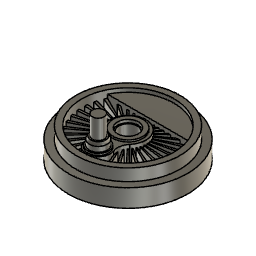
Leading Wheel (Autodesk Fusion 360 design; units mm, degrees)
Autodesk Fusion 360 part; units mm, degrees
sketch "Sketch1" plane through (0, 0, 0) normal (0, 0, 1) x (1, 0, 0) in component "Component"
  circle A0 centre (0, 0) radius 1.55
  circle A1 centre (0, 0) radius 1.75
  circle A2 centre (0, 0) radius 2.5
  circle A3 centre (0, 0) radius 10
  circle A4 centre (0, 0) radius 8.75
  arc A5 (2.2613, -1.9714) -> (1.8622, -4.2706) centre (3.9573, -3.45) ccw
  arc A6 (-1.8622, -4.2706) -> (-2.2613, -1.9714) centre (-3.9573, -3.45) ccw
  circle A7 centre (0, 0) radius 7.75
  arc A8 (2.2613, -1.9714) -> (-2.2613, -1.9714) centre (0, 0) ccw
  arc A9 (-1.8622, -4.2706) -> (1.8622, -4.2706) centre (0, -5) ccw
  line L0 (-0.1744, 2.9949) -> (-0.2026, 3.4782)
  line L1 (-0.3483, 2.9797) -> (-0.4065, 3.4782)
  line L2 (-0.6918, 2.9191) -> (-0.8243, 3.4782)
  line L3 (-0.8604, 2.874) -> (-1.0413, 3.4782)
  line L4 (-1.1882, 2.7546) -> (-1.5003, 3.4782)
  line L5 (-1.3464, 2.6809) -> (-1.7468, 3.4782)
  line L6 (-1.6485, 2.5065) -> (-2.2876, 3.4782)
  line L7 (-1.7915, 2.4064) -> (-2.5894, 3.4782)
  line L8 (-2.0587, 2.1821) -> (-3.2815, 3.4782)
  line L9 (-2.1821, 2.0587) -> (-3.6867, 3.4782)
  line L10 (-2.4064, 1.7915) -> (-4.672, 3.4782)
  line L11 (-2.5065, 1.6485) -> (-5.2883, 3.4782)
  line L12 (-2.6809, 1.3464) -> (-6.9257, 3.4782)
  line L13 (-2.7546, 1.1882) -> (-7.1162, 3.0696)
  line L14 (-2.874, 0.8604) -> (-7.4244, 2.2227)
  line L15 (-2.9191, 0.6918) -> (-7.5411, 1.7873)
  line L16 (-2.9797, 0.3483) -> (-7.6976, 0.8997)
  line L17 (-2.9949, 0.1744) -> (-7.7369, 0.4506)
  line L18 (-2.9949, -0.1744) -> (-7.7369, -0.4506)
  line L19 (-2.9797, -0.3483) -> (-7.6976, -0.8997)
  line L20 (-2.9191, -0.6918) -> (-7.5411, -1.7873)
  line L21 (-2.874, -0.8604) -> (-7.4244, -2.2227)
  line L22 (-2.7546, -1.1882) -> (-7.1162, -3.0696)
  line L23 (-2.6809, -1.3464) -> (-6.9257, -3.4782)
  line L24 (-2.5065, -1.6485) -> (-6.475, -4.2587)
  line L25 (-2.4064, -1.7915) -> (-6.2165, -4.628)
  line L26 (-2.1861, -2.0624) -> (-5.6371, -5.3184)
  line L27 (-2.082, -2.2067) -> (-5.3184, -5.6371)
  line L28 (-1.8963, -2.5472) -> (-4.628, -6.2165)
  line L29 (-1.8156, -2.7604) -> (-4.2587, -6.475)
  line L30 (-1.7078, -3.4005) -> (-3.4782, -6.9257)
  line L31 (-1.9291, -4.4721) -> (-3.0696, -7.1162)
  line L32 (-1.7736, -5.9243) -> (-2.2227, -7.4244)
  line L33 (-1.4989, -6.3242) -> (-1.7873, -7.5411)
  line L34 (-0.7987, -6.8336) -> (-0.8997, -7.6976)
  line L35 (-0.4053, -6.9585) -> (-0.4506, -7.7369)
  line L36 (0.4053, -6.9585) -> (0.4506, -7.7369)
  line L37 (0.7987, -6.8336) -> (0.8997, -7.6976)
  line L38 (1.4989, -6.3242) -> (1.7873, -7.5411)
  line L39 (1.7736, -5.9243) -> (2.2227, -7.4244)
  line L40 (1.9291, -4.4721) -> (3.0696, -7.1162)
  line L41 (1.7078, -3.4005) -> (3.4782, -6.9257)
  line L42 (1.8156, -2.7604) -> (4.2587, -6.475)
  line L43 (1.8963, -2.5472) -> (4.628, -6.2165)
  line L44 (2.082, -2.2067) -> (5.3184, -5.6371)
  line L45 (2.1861, -2.0624) -> (5.6371, -5.3184)
  line L46 (2.4064, -1.7915) -> (6.2165, -4.628)
  line L47 (2.5065, -1.6485) -> (6.475, -4.2587)
  line L48 (2.6809, -1.3464) -> (6.9257, -3.4782)
  line L49 (2.7546, -1.1882) -> (7.1162, -3.0696)
  line L50 (2.874, -0.8604) -> (7.4244, -2.2227)
  line L51 (2.9191, -0.6918) -> (7.5411, -1.7873)
  line L52 (2.9797, -0.3483) -> (7.6976, -0.8997)
  line L53 (2.9949, -0.1744) -> (7.7369, -0.4506)
  line L54 (2.9949, 0.1744) -> (7.7369, 0.4506)
  line L55 (2.9797, 0.3483) -> (7.6976, 0.8997)
  line L56 (2.9191, 0.6918) -> (7.5411, 1.7873)
  line L57 (2.874, 0.8604) -> (7.4244, 2.2227)
  line L58 (2.7546, 1.1882) -> (7.1162, 3.0696)
  line L59 (2.6809, 1.3464) -> (6.9257, 3.4782)
  line L60 (2.5065, 1.6485) -> (5.2883, 3.4782)
  line L61 (2.4064, 1.7915) -> (4.672, 3.4782)
  line L62 (2.1821, 2.0587) -> (3.6867, 3.4782)
  line L63 (2.0587, 2.1821) -> (3.2815, 3.4782)
  line L64 (1.7915, 2.4064) -> (2.5894, 3.4782)
  line L65 (1.6485, 2.5065) -> (2.2876, 3.4782)
  line L66 (1.3464, 2.6809) -> (1.7468, 3.4782)
  line L67 (1.1882, 2.7546) -> (1.5003, 3.4782)
  line L68 (0.8604, 2.874) -> (1.0413, 3.4782)
  line L69 (0.6918, 2.9191) -> (0.8243, 3.4782)
  line L70 (0.3483, 2.9797) -> (0.4065, 3.4782)
  line L71 (0.1744, 2.9949) -> (0.2026, 3.4782)
  circle A10 centre (0, -5) radius 1.75
  circle A11 centre (0, -5) radius 1.5
  circle A12 centre (0, -5) radius 1.25
  circle A13 centre (0, -5) radius 1
  line L72 (-6.9257, 3.4782) -> (6.9257, 3.4782)
  dimension "d1" = 3.1
  dimension "d2" = 3.5
  dimension "d3" = 5
  dimension "d4" = 6
  dimension "d5" = 4
  dimension "d6" = 20
  dimension "d7" = 17.5
  dimension "d8" = 4.5
  dimension "d9" = 4.5
  dimension "d10" = 5
  dimension "d11" = 15.5
  dimension "d15" = 3.5
  dimension "d16" = 3
  dimension "d17" = 2.5
  dimension "d18" = 2
  constraint coincident A0.centre A1.centre
  constraint concentric A0 A1
  constraint concentric A1 A2
  constraint concentric A0 A8
  constraint concentric A3 A8
  constraint tangent A6 A8
  constraint tangent A6 A9
  constraint tangent A5 A8
  constraint tangent A5 A9
  constraint concentric A4 A7
  constraint coincident A8 L0.start
  constraint coincident A8 L1.start
  constraint coincident A8 L3.start
  constraint coincident A8 L2.start
  constraint coincident A8 L5.start
  constraint coincident A8 L4.start
  constraint coincident A8 L6.start
  constraint coincident A8 L7.start
  constraint coincident A8 L8.start
  constraint coincident A8 L9.start
  constraint coincident A8 L10.start
  constraint coincident A8 L11.start
  constraint coincident A8 L12.start
  constraint coincident A8 L13.start
  constraint coincident A8 L14.start
  constraint coincident A8 L15.start
  constraint coincident A8 L16.start
  constraint coincident A8 L17.start
  constraint coincident A8 L19.start
  constraint coincident A8 L18.start
  constraint coincident A8 L20.start
  constraint coincident A8 L21.start
  constraint coincident A8 L22.start
  constraint coincident A8 L23.start
  constraint coincident A8 L24.start
  constraint coincident A8 L25.start
  constraint coincident A6 L26.start
  constraint coincident A6 L27.start
  constraint coincident A6 L28.start
  constraint coincident A6 L29.start
  constraint coincident A6 L30.start
  constraint coincident A9 L31.start
  constraint coincident A9 L32.start
  constraint coincident A9 L33.start
  constraint coincident A9 L34.start
  constraint coincident A9 L35.start
  constraint coincident A9 L36.start
  constraint coincident A9 L37.start
  constraint coincident A9 L38.start
  constraint coincident A9 L39.start
  constraint coincident A9 L40.start
  constraint coincident A5 L41.start
  constraint coincident A5 L42.start
  constraint coincident A5 L43.start
  constraint coincident A5 L44.start
  constraint coincident A5 L45.start
  constraint coincident A8 L46.start
  constraint coincident A8 L47.start
  constraint coincident A8 L48.start
  constraint coincident A8 L49.start
  constraint coincident A8 L50.start
  constraint coincident A8 L51.start
  constraint coincident A8 L52.start
  constraint coincident A8 L53.start
  constraint coincident A8 L54.start
  constraint coincident A8 L55.start
  constraint coincident A8 L56.start
  constraint coincident A8 L57.start
  constraint coincident A8 L58.start
  constraint coincident A8 L59.start
  constraint coincident A8 L60.start
  constraint coincident A8 L61.start
  constraint coincident A8 L62.start
  constraint coincident A8 L63.start
  constraint coincident A8 L64.start
  constraint coincident A8 L65.start
  constraint coincident A8 L66.start
  constraint coincident A8 L67.start
  constraint coincident A8 L68.start
  constraint coincident A8 L69.start
  constraint coincident A8 L70.start
  constraint coincident A8 L71.start
  constraint concentric A9 A10
  constraint concentric A10 A11
  constraint concentric A11 A12
  constraint concentric A12 A13
  constraint horizontal L72
  constraint coincident L59 L72.end
  constraint coincident A7 L59.end
  constraint coincident L72 L11.end
  constraint coincident L72 L10.end
  constraint coincident L72 L9.end
  constraint coincident L72 L7.end
  constraint coincident L72 L6.end
  constraint coincident L72 L8.end
  constraint coincident L72 L5.end
  constraint coincident L72 L3.end
  constraint coincident L72 L0.end
  constraint coincident L72 L70.end
  constraint coincident L72 L4.end
  constraint coincident L72 L2.end
  constraint coincident L72 L1.end
  constraint coincident L72 L71.end
  constraint coincident L72 L67.end
  constraint coincident L72 L66.end
  constraint coincident L72 L65.end
  constraint coincident L72 L64.end
  constraint coincident L72 L63.end
  constraint coincident L72 L62.end
  constraint coincident L72 L61.end
  constraint coincident L72 L60.end
  constraint coincident L72 L68.end
  constraint coincident L72 L69.end
  measures "d1" diameter of A0
  measures "d2" diameter of A1
  measures "d3" diameter of A2
  measures "d4" diameter of A8
  measures "d5" diameter of A9
  measures "d6" diameter of A3
  measures "d7" diameter of A4
  measures "d8" diameter of A6
  measures "d9" diameter of A5
  measures "d10" distance of A0.centre A9.centre
  measures "d11" diameter of A7
  measures "d15" diameter of A10
  measures "d16" diameter of A11
  measures "d17" diameter of A12
  measures "d18" diameter of A13
extrude "Extrude1" add sketch "Sketch1" along normal blind 3 contours A3 makes body 1 in component "Component"
extrude "Extrude2" add sketch "Sketch1" along normal blind 5 contours A4 bodies 1 in component "Component"
extrude "Extrude3" add sketch "Sketch1" along normal blind 4.35 contours A7 L72 bodies 1 in component "Component"
extrude "Extrude4" cut sketch "Sketch1" along normal blind 0.65 contours A7 L72 bodies 1 in component "Component"
extrude "Extrude5" add sketch "Sketch1" along normal blind 4.35 separate body contours A5 A6 A8 A9 makes body 2 in component "Component"
extrude "Extrude6" add sketch "Sketch1" along normal blind 4.65 contours A2 bodies 2 in component "Component"
extrude "Extrude7" add sketch "Sketch1" along normal blind 4.15 contours A1 bodies 2 in component "Component"
extrude "Extrude8" add sketch "Sketch1" along normal blind 4.65 contours A10 bodies 2 in component "Component"
extrude "Extrude9" add sketch "Sketch1" along normal blind 6 separate body contours A13 makes body 3 in component "Component"
extrude "Extrude10" add sketch "Sketch1" along normal blind 9.25 contours A13 bodies 3 in component "Component"
extrude "Extrude11" add sketch "Sketch1" along normal blind 6 contours A12 bodies 3 in component "Component"
extrude "Extrude12" add sketch "Sketch1" along normal blind 5.5 contours A11 bodies 2 3 in component "Component"
extrude "Extrude13" add sketch "Sketch1" along normal blind 3.75 contours A5 A7 L44 L45 | A7 A8 L46 L47 | A5 A7 L42 L43 | A7 A8 L48 L49 | A5 A7 A9 L40 L41 | A7 A8 L50 L51 | A7 A8 L52 L53 | A7 A9 L38 L39 | A7 A8 L54 L55 | A7 A9 L36 L37 | A7 A8 L56 L57 | A7 A9 L34 L35 | A7 A8 L58 L59 | A7 A9 L32 L33 | A8 L60 L61 L72 | A6 A7 A9 L30 L31 | A7 A8 L12 L13 | A8 L62 L63 L72 | A8 L10 L11 L72 | A6 A7 L28 L29 | A7 A8 L14 L15 | A8 L64 L65 L72 | A8 L8 L9 L72 | A6 A7 L26 L27 | A7 A8 L16 L17 | A8 L66 L67 L72 | A8 L6 L7 L72 | A7 A8 L24 L25 | A7 A8 L18 L19 | A8 L68 L69 L72 | A8 L4 L5 L72 | A7 A8 L22 L23 | A7 A8 L20 L21 | A8 L70 L71 L72 | A8 L2 L3 L72 | A8 L0 L1 L72 bodies 1 2 in component "Component"
extrude "Extrude14" cut sketch "Sketch1" along normal blind 1.25 contours A5 A7 L44 L45 | A7 A8 L46 L47 | A5 A7 L42 L43 | A7 A8 L48 L49 | A5 A7 A9 L40 L41 | A7 A8 L50 L51 | A7 A8 L52 L53 | A7 A9 L38 L39 | A7 A8 L54 L55 | A7 A9 L36 L37 | A7 A8 L56 L57 | A7 A9 L34 L35 | A7 A8 L58 L59 | A7 A9 L32 L33 | A8 L60 L61 L72 | A6 A7 A9 L30 L31 | A7 A8 L12 L13 | A8 L62 L63 L72 | A8 L10 L11 L72 | A6 A7 L28 L29 | A7 A8 L14 L15 | A8 L64 L65 L72 | A8 L8 L9 L72 | A6 A7 L26 L27 | A7 A8 L16 L17 | A8 L66 L67 L72 | A8 L6 L7 L72 | A7 A8 L24 L25 | A7 A8 L18 L19 | A8 L68 L69 L72 | A8 L4 L5 L72 | A7 A8 L22 L23 | A7 A8 L20 L21 | A8 L70 L71 L72 | A8 L2 L3 L72 | A8 L0 L1 L72 bodies 1 in component "Component"
fillet "Fillet1" radius 0.8 1 edges at (-1.1654, -4.548, 5.5) on bodies 1 in component "Component"
component "Component" placed x (1, 0, 0) y (0, 1, 0) z (0, 0, 1) at (0, 0, 0)
